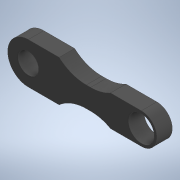
# Autodesk Inventor part: PLEUEL short new
Saved by Autodesk Inventor 2022 (Build 260153000, 153)
## iProperties
Created: 2020-07-02
Part Number: PLEUEL short new
Material: Generic
Document SubType Name: Modeling
Designer: Smit Ambardekar
Density: 1 g/cm^3
Appearance: Generic
Author: Smit Ambardekar
Autodesk Inventor part; units mm, degrees
ref_plane "YZ Plane" through (0, 0, 0) normal (1, 0, 0) x (0, 1, 0)
ref_plane "XZ Plane" through (0, 0, 0) normal (0, 1, 0) x (-1, 0, 0)
ref_plane "XY Plane" through (0, 0, 0) normal (0, 0, 1) x (1, 0, 0)
sketch "Sketch1" plane through (0, 0, 0) normal (0, 0, 1) x (1, 0, 0)
  circle A0 centre (0, 0) radius 4
  circle A1 centre (0, 0) radius 2
  line L0 (0, -4) -> (6, -4)
  line L1 (6, -4) -> (6, 4)
  line L2 (6, 4) -> (0, 4)
  circle A2 centre (22, 0) radius 2.5
  circle A3 centre (22, 0) radius 3
  line L3 (22, -3) -> (16, -3)
  line L4 (16, -3) -> (16, 3)
  line L5 (16, 3) -> (22, 3)
  line L6 (16, -2) -> (6, -2)
  line L7 (6, 2) -> (16, 2)
  dimension "d0" = 8
  dimension "d1" = 4
  dimension "d8" = 6
  dimension "d9" = 5
  dimension "d10" = 6
  dimension "d11" = 6
  dimension "d12" = 6
  dimension "d17" = 10
  dimension "d19" = 4
  constraints: 16 end point, 4 centre point, 4 point on circle, 4 point on line, 3 coincident, 3 tangent, 2 horizontal, 2 perpendicular, 1 parallel
  measures "d0" diameter of A0
  measures "d1" diameter of A1
  measures "d8" distance of L0.start L0.end
  measures "d9" diameter of A2
  measures "d10" diameter of A3
  measures "d11" distance of L3.start L3.end
  measures "d12" distance of L3.end L4.end
  measures "d17" distance between parallel lines of L4 L1
  measures "d19" distance of L6.start L7.end
extrude "Extrusion1" add sketch "Sketch1" along normal blind 3
fillet "Fillet1" radius 8 1 edges at (6, -2, 1.5)
fillet "Fillet2" radius 8 3 edges at (6, 2, 1.5) (16, 2, 1.5) (16, -2, 1.5)
body "Solid1"
